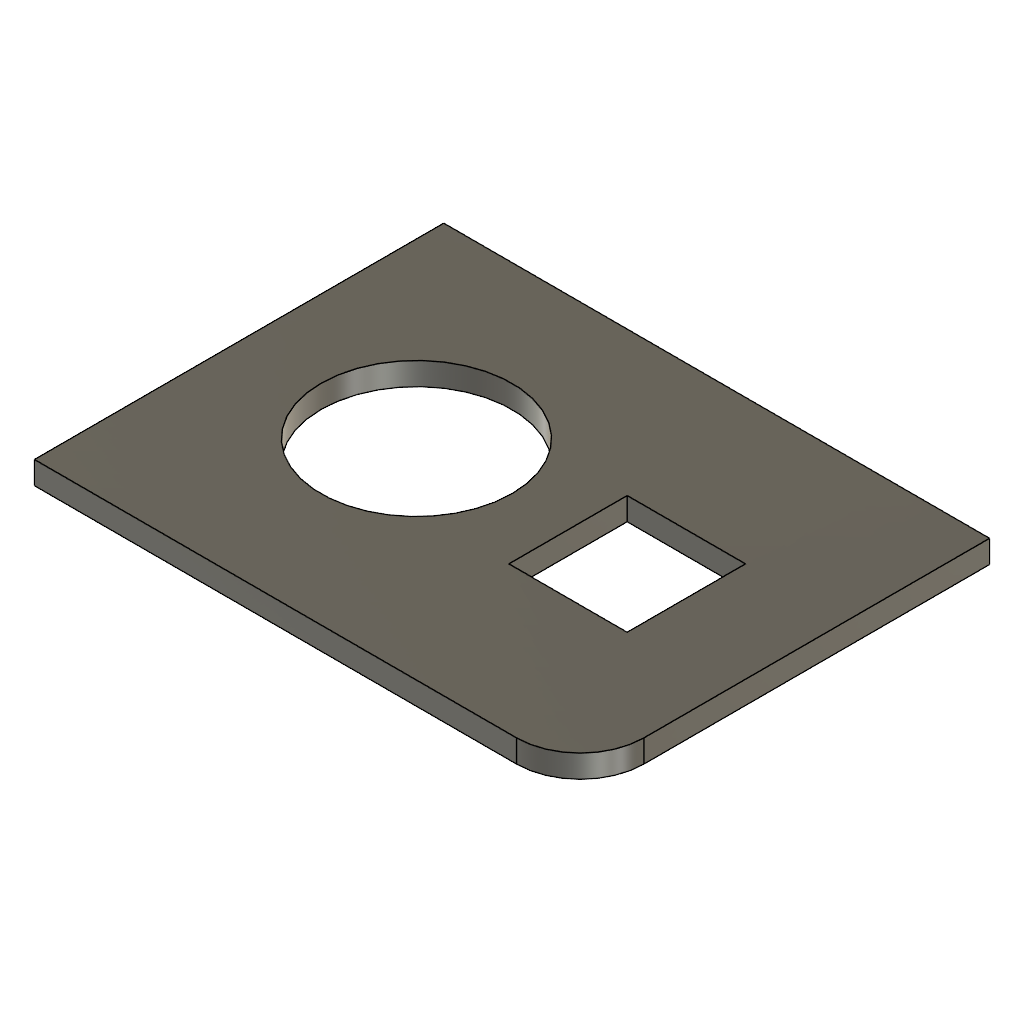
tuile-couleur (Autodesk Fusion 360 design; units mm, degrees)
part number: 2026-10-04-18-01-57-622
Autodesk Fusion 360 part; units mm, degrees
sketch "Esquisse1" plane through (0, 0, 0) normal (0, 0, 1) x (1, 0, 0)
  line L0 (0, 0) -> (60, 0)
  line L1 (60, 0) -> (60, 45)
  line L2 (60, 45) -> (0, 45)
  line L3 (0, 45) -> (0, 0)
  dimension "d1" = 60
  dimension "d2" = 45
  constraint horizontal L0
  constraint vertical L1
  constraint horizontal L2
  constraint vertical L3
  constraint coincident L0.start L3.end
  measures "d1" distance of L0.start L0.end
  measures "d2" distance of L0.start L2.end
extrude "Extrusion1" add sketch "Esquisse1" along normal blind 2.5
fillet "Congé1" radius 7 1 edges at (60, 0, 1.25)
sketch "Esquisse2" plane through (0, 0, 2.5) normal (0, 0, 1) x (-1, 0, 0)
  arc A0 (-53, 0) -> (-60, -7) centre (-53, -7) ccw
  line L0 (-60, -7) -> (-60, -45)
  line L1 (-60, -45) -> (0, -45)
  line L2 (0, -45) -> (0, 0)
  line L3 (0, 0) -> (-53, 0)
  line L4 (-36.0159, -29.1423) -> (-49.0159, -29.1423)
  line L5 (-49.0159, -29.1423) -> (-49.0159, -16.1423)
  line L6 (-49.0159, -16.1423) -> (-36.0159, -16.1423)
  line L7 (-36.0159, -16.1423) -> (-36.0159, -29.1423)
  dimension "d7" = 13
  dimension "d8" = 13
  constraint horizontal L4
  constraint vertical L5
  constraint horizontal L6
  constraint vertical L7
  measures "d7" distance of L4.start L4.end
  measures "d8" distance of L4.start L6.end
extrude "Extrusion2" cut sketch "Esquisse2" against normal blind 2.5 contours L4 L5 L6 L7
sketch "Esquisse3" plane through (0, 0, 2.5) normal (0, 0, 1) x (-1, 0, 0)
  line L0 (-49.0159, -29.1423) -> (-49.0159, -16.1423)
  line L1 (-49.0159, -16.1423) -> (-36.0159, -16.1423)
  line L2 (-36.0159, -16.1423) -> (-36.0159, -29.1423)
  line L3 (-36.0159, -29.1423) -> (-49.0159, -29.1423)
  arc A0 (-53, 0) -> (-60, -7) centre (-53, -7) ccw
  line L4 (-60, -7) -> (-60, -45)
  line L5 (-60, -45) -> (0, -45)
  line L6 (0, -45) -> (0, 0)
  line L7 (0, 0) -> (-53, 0)
  circle A1 centre (-19, -23) radius 10.5
  dimension "d11" = 21
  measures "d11" diameter of A1
extrude "Extrusion3" cut sketch "Esquisse3" against normal blind 2.5 contours A1
